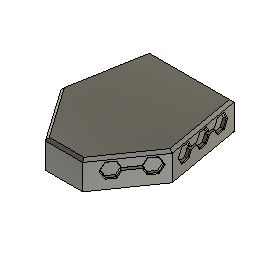
wedge_10deg_50mm (Autodesk Fusion 360 design; units mm, degrees)
Autodesk Fusion 360 part; units mm, degrees
sketch "case_bottom" plane through (0, 0, 0) normal (0, 0, 1) x (1, 0, 0)
  line L0 (-35.1064, -29.6171) -> (-72.9833, -15.1643)
  line L1 (-72.9833, -15.1643) -> (-73.0723, -15.1303)
  line L2 (-112.846, -13.2641) -> (-134.2997, -22.0522)
  line L3 (-148.4991, -102.5811) -> (-32.4939, -123.0359)
  line L4 (-42.7749, -73.1075) -> (-35.1064, -29.6171)
  line L5 (-73.0723, -15.1303) -> (-91.9987, -11.7931)
  line L6 (-134.2997, -22.0522) -> (-148.4991, -102.5811)
  line L7 (-32.4939, -123.0359) -> (-21.325, -103.6908)
  line L8 (-21.325, -103.6908) -> (-42.7749, -73.1075)
  line L9 (-91.9987, -11.7931) -> (-112.846, -13.2641)
  line L10 (-39.6045, -72.4034) -> (-31.7216, -27.6976)
  line L11 (-72.2698, -12.2255) -> (-91.8415, -8.7745)
  line L12 (-136.967, -19.9029) -> (-151.9745, -105.0146)
  line L13 (-17.7705, -103.5343) -> (-39.6045, -72.4034)
  line L14 (-91.8415, -8.7745) -> (-113.5376, -10.3054)
  line L15 (-113.5376, -10.3054) -> (-136.967, -19.9029)
  line L16 (-30.9462, -126.3551) -> (-17.7705, -103.5343)
  line L17 (-151.9745, -105.0146) -> (-30.9462, -126.3551)
  line L18 (-31.7216, -27.6976) -> (-72.2698, -12.2255)
  line L19 (-91.9358, -10.5856) -> (-113.1226, -12.0806)
  line L20 (-33.7525, -28.8493) -> (-72.7513, -13.9684)
  line L21 (-72.7513, -13.9684) -> (-91.9358, -10.5856)
  line L22 (-41.5067, -72.8258) -> (-33.7525, -28.8493)
  line L23 (-149.8893, -103.5545) -> (-31.8748, -124.3636)
  line L24 (-19.9032, -103.6282) -> (-41.5067, -72.8258)
  line L25 (-113.1226, -12.0806) -> (-135.3666, -21.1925)
  line L26 (-135.3666, -21.1925) -> (-149.8893, -103.5545)
  line L27 (-31.8748, -124.3636) -> (-19.9032, -103.6282)
  line L28 (-135.9001, -20.7626) -> (-150.5844, -104.0412)
  line L29 (-113.261, -11.4889) -> (-135.9001, -20.7626)
  line L30 (-150.5844, -104.0412) -> (-31.5653, -125.0275)
  line L31 (-19.1923, -103.5969) -> (-40.8727, -72.685)
  line L32 (-33.0755, -28.4654) -> (-72.3416, -13.4825)
  line L33 (-40.8727, -72.685) -> (-33.0755, -28.4654)
  line L34 (-91.9044, -9.9819) -> (-113.261, -11.4889)
  line L35 (-31.5653, -125.0275) -> (-19.1923, -103.5969)
  line L36 (-72.5908, -13.3874) -> (-91.9044, -9.9819)
  line L37 (-72.3416, -13.4825) -> (-72.5908, -13.3874)
  circle A0 centre (-112.6416, -34.5542) radius 2.2
  circle A1 centre (-119.2403, -71.9769) radius 2.2
  circle A2 centre (-61.4316, -43.5839) radius 2.2
  circle A3 centre (-53.1512, -89.5442) radius 2.2
  line L38 (-110.3652, -87.8695) -> (-142.8638, -82.1391)
  line L39 (-113.4908, -105.5961) -> (-110.3652, -87.8695)
  line L40 (-142.8638, -82.1391) -> (-145.9895, -99.8657)
  line L41 (-145.9895, -99.8657) -> (-113.4908, -105.5961)
  line L42 (-109.5644, -103.628) -> (-110.5803, -109.3891)
  line L43 (-101.914, -110.9172) -> (-100.8981, -105.1561)
  line L44 (-100.8981, -105.1561) -> (-109.5644, -103.628)
  line L45 (-99.0995, -106.4734) -> (-99.7073, -109.9202)
  line L46 (-90.844, -111.4831) -> (-90.2363, -108.0362)
  line L47 (-99.7073, -109.9202) -> (-90.844, -111.4831)
  line L48 (-90.2363, -108.0362) -> (-99.0995, -106.4734)
  line L49 (-38.2759, -97.5309) -> (-30.8216, -92.3113)
  line L50 (-44.5852, -88.5202) -> (-38.2759, -97.5309)
  line L51 (-30.8216, -92.3113) -> (-37.1309, -83.3007)
  line L52 (-37.1309, -83.3007) -> (-44.5852, -88.5202)
  line L53 (-108.5664, -75.9406) -> (-117.0358, -74.4473)
  line L54 (-117.0358, -74.4473) -> (-118.5812, -83.2121)
  line L55 (-118.5812, -83.2121) -> (-110.1119, -84.7054)
  line L56 (-110.1119, -84.7054) -> (-108.5664, -75.9406)
  line L57 (-6.7216, 0) -> (-6.7216, -133.1408) construction
  line L58 (24.8326, -97.5309) -> (17.3783, -92.3113)
  line L59 (58.8265, -12.2255) -> (78.3982, -8.7745)
  line L60 (19.0506, -123.0359) -> (7.8817, -103.6908)
  line L61 (28.0634, -72.8258) -> (20.3092, -28.8493)
  line L62 (-6.7216, 0) -> (-6.7216, -133.1408) construction
  line L63 (58.8983, -13.4825) -> (59.1475, -13.3874)
  line L64 (18.122, -125.0275) -> (5.749, -103.5969)
  line L65 (27.4294, -72.685) -> (19.6322, -28.4654)
  circle A4 centre (105.797, -71.9769) radius 2.2
  line L66 (18.2784, -27.6976) -> (58.8265, -12.2255)
  line L67 (96.6686, -84.7054) -> (95.1231, -75.9406)
  line L68 (17.5029, -126.3551) -> (4.3272, -103.5343)
  line L69 (105.1379, -83.2121) -> (96.6686, -84.7054)
  line L70 (26.1612, -72.4034) -> (18.2784, -27.6976)
  line L71 (103.5925, -74.4473) -> (105.1379, -83.2121)
  circle A5 centre (47.9883, -43.5839) radius 2.2
  line L72 (87.4548, -105.1561) -> (96.1211, -103.628)
  line L73 (19.6322, -28.4654) -> (58.8983, -13.4825)
  line L74 (76.793, -108.0362) -> (85.6562, -106.4734)
  line L75 (5.749, -103.5969) -> (27.4294, -72.685)
  line L76 (78.3982, -8.7745) -> (100.0943, -10.3054)
  line L77 (88.4707, -110.9172) -> (87.4548, -105.1561)
  line L78 (99.8177, -11.4889) -> (122.4568, -20.7626)
  line L79 (100.0475, -105.5961) -> (96.9219, -87.8695)
  line L80 (95.1231, -75.9406) -> (103.5925, -74.4473)
  line L81 (96.1211, -103.628) -> (97.137, -109.3891)
  line L82 (132.5462, -99.8657) -> (100.0475, -105.5961)
  circle A6 centre (99.1983, -34.5542) radius 2.2
  line L83 (96.9219, -87.8695) -> (129.4205, -82.1391)
  line L84 (120.8564, -22.0522) -> (135.0558, -102.5811)
  line L85 (121.9234, -21.1925) -> (136.446, -103.5545)
  line L86 (4.3272, -103.5343) -> (26.1612, -72.4034)
  line L87 (86.264, -109.9202) -> (77.4007, -111.4831)
  line L88 (6.4599, -103.6282) -> (28.0634, -72.8258)
  line L89 (100.0943, -10.3054) -> (123.5237, -19.9029)
  line L90 (77.4007, -111.4831) -> (76.793, -108.0362)
  line L91 (18.4315, -124.3636) -> (6.4599, -103.6282)
  line L92 (78.4925, -10.5856) -> (99.6793, -12.0806)
  line L93 (85.6562, -106.4734) -> (86.264, -109.9202)
  line L94 (78.4611, -9.9819) -> (99.8177, -11.4889)
  line L95 (135.0558, -102.5811) -> (19.0506, -123.0359)
  line L96 (99.4027, -13.2641) -> (120.8564, -22.0522)
  line L97 (31.1419, -88.5202) -> (24.8326, -97.5309)
  line L98 (129.4205, -82.1391) -> (132.5462, -99.8657)
  line L99 (59.54, -15.1643) -> (59.629, -15.1303)
  line L100 (21.6631, -29.6171) -> (59.54, -15.1643)
  line L101 (122.4568, -20.7626) -> (137.1411, -104.0412)
  circle A7 centre (39.7079, -89.5442) radius 2.2
  line L102 (29.3316, -73.1075) -> (21.6631, -29.6171)
  line L103 (23.6877, -83.3007) -> (31.1419, -88.5202)
  line L104 (99.6793, -12.0806) -> (121.9234, -21.1925)
  line L105 (7.8817, -103.6908) -> (29.3316, -73.1075)
  line L106 (17.3783, -92.3113) -> (23.6877, -83.3007)
  line L107 (123.5237, -19.9029) -> (138.5312, -105.0146)
  line L108 (137.1411, -104.0412) -> (18.122, -125.0275)
  line L109 (59.629, -15.1303) -> (78.5554, -11.7931)
  line L110 (59.308, -13.9684) -> (78.4925, -10.5856)
  line L111 (136.446, -103.5545) -> (18.4315, -124.3636)
  line L112 (138.5312, -105.0146) -> (17.5029, -126.3551)
  line L113 (59.1475, -13.3874) -> (78.4611, -9.9819)
  line L114 (78.5554, -11.7931) -> (99.4027, -13.2641)
  line L115 (20.3092, -28.8493) -> (59.308, -13.9684)
  line L116 (-31.7216, -27.6976) -> (18.2784, -27.6976)
  line L117 (-17.7705, -103.5343) -> (4.3272, -103.5343)
  dimension "d1" = 25
  dimension "d2" = 25
  constraint vertical L57
  constraint perpendicular L62 L116
  constraint horizontal L117
  measures "d1" distance of L10.end L57
  measures "d2" distance of L66.start L62
extrude "Extrude1" add sketch "case_bottom" along normal blind 16.6 contours L10 L13 L70 L86 L116 L117
sketch "Sketch2" plane through (12.9906, 2.2906, 0) normal (0.984808, 0.173648, 0) x (-0.173648, 0.984808, 0)
  line L0 (-75.8462, 0) -> (-30.4508, 0)
  line L1 (-30.4508, 0) -> (-30.4508, 16.6)
  line L2 (-30.4508, 16.6) -> (-75.8462, 16.6)
  line L3 (-75.8462, 16.6) -> (-75.8462, 0)
  line L4 (-30.4508, 9.7) -> (-75.8462, 9.7) construction
  line L5 (-63.8281, 13.6602) -> (-68.4179, 13.6897)
  line L6 (-68.4179, 13.6897) -> (-70.7384, 9.7295)
  line L7 (-70.7384, 9.7295) -> (-68.469, 5.7398)
  line L8 (-68.469, 5.7398) -> (-63.8791, 5.7103)
  line L9 (-63.8791, 5.7103) -> (-61.5587, 9.6705)
  line L10 (-61.5587, 9.6705) -> (-63.8281, 13.6602)
  line L11 (-50.8281, 13.6602) -> (-55.4179, 13.6897)
  line L12 (-55.4179, 13.6897) -> (-57.7384, 9.7295)
  line L13 (-57.7384, 9.7295) -> (-55.469, 5.7398)
  line L14 (-55.469, 5.7398) -> (-50.8791, 5.7103)
  line L15 (-50.8791, 5.7103) -> (-48.5587, 9.6705)
  line L16 (-48.5587, 9.6705) -> (-50.8281, 13.6602)
  line L17 (-37.8281, 13.6602) -> (-42.4179, 13.6897)
  line L18 (-42.4179, 13.6897) -> (-44.7384, 9.7295)
  line L19 (-44.7384, 9.7295) -> (-42.469, 5.7398)
  line L20 (-42.469, 5.7398) -> (-37.8791, 5.7103)
  line L21 (-37.8791, 5.7103) -> (-35.5587, 9.6705)
  line L22 (-35.5587, 9.6705) -> (-37.8281, 13.6602)
  line L23 (-66.1485, 8.95) -> (-40.1485, 8.95)
  arc A0 (-40.1485, 8.95) -> (-40.1485, 10.45) centre (-40.1485, 9.7) ccw
  line L24 (-40.1485, 10.45) -> (-66.1485, 10.45)
  arc A1 (-66.1485, 10.45) -> (-66.1485, 8.95) centre (-66.1485, 9.7) ccw
  line L25 (-66.1485, 9.7) -> (-40.1485, 9.7) construction
  point P0 (-53.1485, 9.7)
  point P1 (-40.1485, 9.7)
  point P2 (-66.1485, 9.7)
  point P3 (-66.1485, 9.7)
  point P4 (-53.1485, 9.7)
  point P5 (-40.1485, 9.7)
  dimension "d5" = 6.9
  dimension "d6" = 13
  dimension "d7" = 13
  dimension "d8" = 3.975
  dimension "d9" = 3.975
  dimension "d10" = 3.975
  dimension "d11" = 1.5
  constraint coincident L1 L4.start
  constraint coincident L3 L4.end
  constraint perpendicular L3 L4
  constraint midpoint L4 P4
  constraint coincident L4 P5
  constraint coincident L4 P3
  constraint coincident P3 P2
  constraint coincident P4 P0
  constraint coincident P5 P1
  constraint tangent L23 A0
  constraint tangent A0 L24
  constraint parallel L23 L24
  constraint tangent L24 A1
  constraint tangent L23 A1
  constraint parallel L4 L25
  measures "d5" distance of L2 L4
  measures "d6" distance of P4 P3
  measures "d7" distance of P4 P5
  measures "d8" distance of P3 L10
  measures "d9" distance of P4 L16
  measures "d10" distance of P5 L22
  measures "d11" diameter of A0
extrude "Extrude2" cut sketch "Sketch2" against normal blind 2 contours L5 L6 L7 L8 L9 L10 L23 L24 A1 | L9 L10 L12 L13 L23 L24 | L9 L10 L23 L24 A1 | L12 L13 L15 L16 L23 L24 | L11 L12 L16 L24 | L15 L16 L18 L19 L23 L24 | L13 L14 L15 L23 | L18 L19 L23 A0 L24 | L17 L18 L19 L20 L21 L22 L23 A0 L24
sketch "Sketch3" plane through (51.573, -36.1712, 0) normal (0.818709, -0.574209, 0) x (0.574209, 0.818709, 0)
  line L0 (-82.2797, 0) -> (-44.2553, 0)
  line L1 (-44.2553, 0) -> (-44.2553, 16.6)
  line L2 (-44.2553, 16.6) -> (-82.2797, 16.6)
  line L3 (-82.2797, 16.6) -> (-82.2797, 0)
  line L4 (-82.2797, 9.7) -> (-44.2553, 9.7) construction
  line L5 (-67.9848, 13.6751) -> (-72.5747, 13.6749)
  line L6 (-72.5747, 13.6749) -> (-74.8696, 9.6999)
  line L7 (-74.8696, 9.6999) -> (-72.5745, 5.7249)
  line L8 (-72.5745, 5.7249) -> (-67.9846, 5.7251)
  line L9 (-67.9846, 5.7251) -> (-65.6897, 9.7001)
  line L10 (-65.6897, 9.7001) -> (-67.9848, 13.6751)
  line L11 (-56.8452, 9.7001) -> (-54.5503, 5.7251)
  line L12 (-54.5503, 5.7251) -> (-49.9604, 5.7249)
  line L13 (-49.9604, 5.7249) -> (-47.6653, 9.6999)
  line L14 (-47.6653, 9.6999) -> (-49.9602, 13.6749)
  line L15 (-49.9602, 13.6749) -> (-54.5501, 13.6751)
  line L16 (-54.5501, 13.6751) -> (-56.8452, 9.7001)
  line L17 (-52.2553, 10.45) -> (-70.2797, 10.45)
  arc A0 (-70.2797, 10.45) -> (-70.2797, 8.95) centre (-70.2797, 9.7) ccw
  line L18 (-70.2797, 8.95) -> (-52.2553, 8.95)
  arc A1 (-52.2553, 8.95) -> (-52.2553, 10.45) centre (-52.2553, 9.7) ccw
  line L19 (-52.2553, 9.7) -> (-70.2797, 9.7) construction
  point P0 (-70.2797, 9.7)
  point P1 (-52.2553, 9.7)
  point P2 (-70.2797, 9.7)
  point P3 (-52.2553, 9.7)
  dimension "d14" = 6.9
  dimension "d15" = 8
  dimension "d16" = 12
  dimension "d17" = 3.975
  dimension "d18" = 3.975
  dimension "d19" = 1.5
  constraint coincident L3 L4.start
  constraint coincident L1 L4.end
  constraint perpendicular L1 L4
  constraint coincident L4 P2
  constraint coincident L4 P3
  constraint coincident P2 P0
  constraint coincident P3 P1
  constraint tangent L17 A0
  constraint tangent A0 L18
  constraint parallel L17 L18
  constraint tangent L18 A1
  constraint tangent L17 A1
  constraint parallel L4 L19
  measures "d14" distance of L2 L4
  measures "d15" distance of L1 P3
  measures "d16" distance of L3 P2
  measures "d17" distance of P2 L10
  measures "d18" distance of P3 L16
  measures "d19" diameter of A0
extrude "Extrude3" cut sketch "Sketch3" against normal blind 2 contours L5 L6 L7 L8 L9 L10 L17 A0 L18 | L9 L10 L11 L16 L17 L18 | L9 L10 L17 A0 L18 | L11 L16 L17 L18 A1 | L11 L12 L13 L14 L15 L16 L17 L18 A1
sketch "Sketch4" plane through (-60.5838, -42.491, 0) normal (-0.818709, -0.574209, 0) x (0.574209, -0.818709, 0)
  line L0 (36.536, 0) -> (74.5604, 0)
  line L1 (74.5604, 0) -> (74.5604, 16.6)
  line L2 (74.5604, 16.6) -> (36.536, 16.6)
  line L3 (36.536, 16.6) -> (36.536, 0)
  line L4 (74.5604, 9.7) -> (36.536, 9.7) construction
  line L5 (46.8263, 13.6777) -> (42.2364, 13.6723)
  line L6 (42.2364, 13.6723) -> (39.9461, 9.6946)
  line L7 (39.9461, 9.6946) -> (42.2457, 5.7223)
  line L8 (42.2457, 5.7223) -> (46.8356, 5.7277)
  line L9 (46.8356, 5.7277) -> (49.1259, 9.7054)
  line L10 (49.1259, 9.7054) -> (46.8263, 13.6777)
  line L11 (57.9705, 9.7054) -> (60.2608, 5.7277)
  line L12 (60.2608, 5.7277) -> (64.8507, 5.7223)
  line L13 (64.8507, 5.7223) -> (67.1503, 9.6946)
  line L14 (67.1503, 9.6946) -> (64.86, 13.6723)
  line L15 (64.86, 13.6723) -> (60.2701, 13.6777)
  line L16 (60.2701, 13.6777) -> (57.9705, 9.7054)
  line L17 (44.536, 8.95) -> (62.5604, 8.95)
  arc A0 (62.5604, 8.95) -> (62.5604, 10.45) centre (62.5604, 9.7) ccw
  line L18 (62.5604, 10.45) -> (44.536, 10.45)
  arc A1 (44.536, 10.45) -> (44.536, 8.95) centre (44.536, 9.7) ccw
  line L19 (44.536, 9.7) -> (62.5604, 9.7) construction
  point P0 (44.536, 9.7)
  point P1 (62.5604, 9.7)
  point P2 (44.536, 9.7)
  point P3 (62.5604, 9.7)
  dimension "d22" = 6.9
  dimension "d23" = 8
  dimension "d24" = 12
  dimension "d25" = 3.975
  dimension "d26" = 3.975
  dimension "d27" = 1.5
  constraint coincident L1 L4.start
  constraint coincident L3 L4.end
  constraint perpendicular L3 L4
  constraint coincident L4 P2
  constraint coincident L4 P3
  constraint coincident P2 P0
  constraint coincident P3 P1
  constraint tangent L17 A0
  constraint tangent A0 L18
  constraint parallel L17 L18
  constraint tangent L18 A1
  constraint tangent L17 A1
  constraint parallel L4 L19
  measures "d22" distance of L2 L4
  measures "d23" distance of L3 P2
  measures "d24" distance of L1 P3
  measures "d25" distance of P2 L10
  measures "d26" distance of P3 L16
  measures "d27" diameter of A0
extrude "Extrude4" cut sketch "Sketch4" against normal blind 2 contours L5 L6 L7 L8 L9 L10 L17 L18 A1 | L9 L10 L11 L16 L17 L18 | L9 L10 L17 L18 A1 | L11 L16 L17 A0 L18 | L11 L12 L13 L14 L15 L16 L17 A0 L18
sketch "Sketch5" plane through (-26.0286, 4.5895, 0) normal (-0.984808, 0.173648, 0) x (-0.173648, -0.984808, 0)
  line L0 (32.7852, 0) -> (78.1806, 0)
  line L1 (78.1806, 0) -> (78.1806, 16.6)
  line L2 (78.1806, 16.6) -> (32.7852, 16.6)
  line L3 (32.7852, 16.6) -> (32.7852, 0)
  line L4 (32.7852, 9.7) -> (78.1806, 9.7) construction
  line L5 (44.7753, 13.6765) -> (40.1854, 13.6735)
  line L6 (40.1854, 13.6735) -> (37.893, 9.697)
  line L7 (37.893, 9.697) -> (40.1905, 5.7235)
  line L8 (40.1905, 5.7235) -> (44.7805, 5.7265)
  line L9 (44.7805, 5.7265) -> (47.0729, 9.703)
  line L10 (47.0729, 9.703) -> (44.7753, 13.6765)
  line L11 (57.7753, 13.6765) -> (53.1854, 13.6735)
  line L12 (53.1854, 13.6735) -> (50.893, 9.697)
  line L13 (50.893, 9.697) -> (53.1905, 5.7235)
  line L14 (53.1905, 5.7235) -> (57.7805, 5.7265)
  line L15 (57.7805, 5.7265) -> (60.0729, 9.703)
  line L16 (60.0729, 9.703) -> (57.7753, 13.6765)
  line L17 (70.7753, 13.6765) -> (66.1854, 13.6735)
  line L18 (66.1854, 13.6735) -> (63.893, 9.697)
  line L19 (63.893, 9.697) -> (66.1905, 5.7235)
  line L20 (66.1905, 5.7235) -> (70.7805, 5.7265)
  line L21 (70.7805, 5.7265) -> (73.0729, 9.703)
  line L22 (73.0729, 9.703) -> (70.7753, 13.6765)
  line L23 (68.4829, 10.45) -> (42.4829, 10.45)
  arc A0 (42.4829, 10.45) -> (42.4829, 8.95) centre (42.4829, 9.7) ccw
  line L24 (42.4829, 8.95) -> (68.4829, 8.95)
  arc A1 (68.4829, 8.95) -> (68.4829, 10.45) centre (68.4829, 9.7) ccw
  line L25 (68.4829, 9.7) -> (42.4829, 9.7) construction
  point P0 (55.4829, 9.7)
  point P1 (68.4829, 9.7)
  point P2 (42.4829, 9.7)
  point P3 (42.4829, 9.7)
  point P4 (55.4829, 9.7)
  point P5 (68.4829, 9.7)
  dimension "d30" = 6.9
  dimension "d31" = 13
  dimension "d32" = 13
  dimension "d33" = 3.975
  dimension "d34" = 3.975
  dimension "d35" = 3.975
  dimension "d36" = 1.5
  constraint coincident L3 L4.start
  constraint coincident L1 L4.end
  constraint perpendicular L1 L4
  constraint midpoint L4 P4
  constraint coincident L4 P5
  constraint coincident L4 P3
  constraint coincident P3 P2
  constraint coincident P4 P0
  constraint coincident P5 P1
  constraint tangent L23 A0
  constraint tangent A0 L24
  constraint parallel L23 L24
  constraint tangent L24 A1
  constraint tangent L23 A1
  constraint parallel L4 L25
  measures "d30" distance of L2 L4
  measures "d31" distance of P4 P3
  measures "d32" distance of P4 P5
  measures "d33" distance of P3 L10
  measures "d34" distance of P4 L16
  measures "d35" distance of P5 L22
  measures "d36" diameter of A0
extrude "Extrude5" cut sketch "Sketch5" against normal blind 2 contours L5 L6 L7 L8 L9 L10 L23 A0 L24 | L9 L10 L12 L13 L23 L24 | L9 L10 L23 A0 L24 | L12 L13 L15 L16 L23 L24 | L11 L12 L16 L23 | L15 L16 L18 L19 L23 L24 | L13 L14 L15 L24 | L18 L19 L23 L24 A1 | L17 L18 L19 L20 L21 L22 L23 L24 A1
chamfer "Chamfer1" distance 0.4 angle 45 59 edges at (-33.4052, -37.2455, 13.675) (-32.8076, -33.8566, 11.6853) (-32.8081, -33.8591, 7.7103) (-33.4061, -37.2505, 5.725) (-33.9657, -40.4242, 12.0632) (-33.9659, -40.4257, 7.3382) (-35.1028, -46.8728, 12.0618) (-35.6626, -50.048, 13.675) (-36.2231, -53.2267, 12.0632) (-36.2234, -53.2282, 7.3382) (-35.6635, -50.053, 5.725) (-35.103, -46.8743, 7.3368) (-37.3602, -59.6753, 12.0618) (-37.92, -62.8505, 13.675) (-37.3604, -59.6768, 7.3368) (-37.9209, -62.8555, 5.725) (-38.5185, -66.2444, 7.7147) (-38.518, -66.2419, 11.6897) (-36.9888, -76.1328, 11.6835) (-35.0135, -78.9492, 13.675) (-33.1592, -81.593, 12.0638) (-33.1577, -81.5952, 7.3388) (-36.9862, -76.1366, 7.7085) (-26.5126, -91.0698, 12.0638) (-24.6584, -93.7136, 13.675) (-22.683, -96.53, 11.6835) (-22.6857, -96.5262, 7.7085) (-24.6637, -93.7059, 5.725) (-26.5142, -91.0675, 7.3388) (9.241, -96.5282, 11.6874) (9.2411, -96.5281, 7.7124) (11.2178, -93.7097, 5.725) (11.2177, -93.7099, 13.675) (13.0701, -91.0687, 12.0625) (13.0701, -91.0686, 7.3375) (19.7152, -81.5941, 12.0625) (21.5676, -78.9529, 13.675) (19.7151, -81.5942, 7.3375) (21.5674, -78.9531, 5.725) (23.5442, -76.1347, 7.7124) (23.5442, -76.1346, 11.6874) (25.0727, -66.2305, 11.7096) (25.0772, -66.2556, 7.7346) (24.4816, -62.8781, 5.7251) (23.9183, -59.6834, 7.3302) (23.9157, -59.6687, 12.0551) (24.4728, -62.8279, 13.6749) (22.7787, -53.2201, 12.0698) (22.7812, -53.2348, 7.3449) (22.2242, -50.0756, 5.7251) (21.6609, -46.8809, 7.3302) (21.6583, -46.8662, 12.0551) (22.2153, -50.0254, 13.6749) (20.5212, -40.4176, 12.0698) (20.5238, -40.4323, 7.3449) (19.9668, -37.2731, 5.7251) (19.3668, -33.8705, 7.6904) (19.3624, -33.8453, 11.6654) (19.9579, -37.2229, 13.6749)
chamfer "Chamfer2" distance 1.5 angle 45 1 faces at (1.6117, -57.5014, 16.6)
